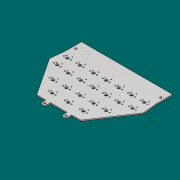
# Autodesk Inventor part: pcb_v2
Saved by Autodesk Inventor 2018 (Build 220112000, 112)
## iProperties
Created: 2021-07-30
Part Number: pcb_v2
Material: アルミニウム 6061
Document SubType Name: Modeling
Designer: gisen
Density: 2.7 g/cm^3
Appearance: アルミニウム - フラット
Author: gisen
Autodesk Inventor part; units mm, degrees
(part 1 of 2)
ref_plane "YZ Plane" through (0, 0, 0) normal (1, 0, 0) x (0, 1, 0)
ref_plane "XZ Plane" through (0, 0, 0) normal (0, 1, 0) x (-1, 0, 0)
ref_plane "XY Plane" through (0, 0, 0) normal (0, 0, 1) x (1, 0, 0)
sketch "スケッチ1" plane through (0, 0, 0) normal (0, 0, 1) x (1, 0, 0)
  line L0 (8.89, 54.5206) -> (46.4896, -2.286)
  arc A0 (46.4844, -2.2894) -> (46.4948, -2.2826) centre (46.4896, -2.286) ccw
  arc A1 (8.8952, 54.524) -> (8.8848, 54.5171) centre (8.89, 54.5206) ccw
  line L1 (150.2689, 54.5206) -> (112.6693, -2.286)
  arc A2 (112.6641, -2.2826) -> (112.6745, -2.2894) centre (112.6693, -2.286) ccw
  arc A3 (150.2742, 54.5171) -> (150.2637, 54.524) centre (150.269, 54.5206) ccw
  line L2 (147.988, 100.33) -> (11.1709, 100.33)
  arc A4 (11.1709, 100.3362) -> (11.1709, 100.3238) centre (11.1709, 100.33) ccw
  arc A5 (147.988, 100.3238) -> (147.988, 100.3362) centre (147.988, 100.33) ccw
  line L3 (11.1709, 100.33) -> (11.1709, 76.8708)
  arc A6 (11.1647, 76.8708) -> (11.1772, 76.8708) centre (11.1709, 76.8708) ccw
  arc A7 (11.1772, 100.33) -> (11.1647, 100.33) centre (11.1709, 100.33) ccw
  line L4 (8.89, 54.5206) -> (11.1709, 76.8708)
  arc A8 (11.1771, 76.8701) -> (11.1647, 76.8714) centre (11.1709, 76.8707) ccw
  arc A9 (8.8838, 54.5212) -> (8.8962, 54.5199) centre (8.89, 54.5206) ccw
  line L5 (150.2689, 54.5206) -> (147.988, 76.8708)
  arc A10 (147.9942, 76.8714) -> (147.9818, 76.8701) centre (147.988, 76.8707) ccw
  arc A11 (150.2627, 54.5199) -> (150.2752, 54.5212) centre (150.269, 54.5206) ccw
  line L6 (147.988, 100.33) -> (147.988, 76.8708)
  arc A12 (147.9818, 76.8708) -> (147.9943, 76.8708) centre (147.988, 76.8708) ccw
  arc A13 (147.9943, 100.33) -> (147.9818, 100.33) centre (147.988, 100.33) ccw
  line L7 (147.988, 76.8708) -> (150.2689, 54.5435)
  arc A14 (150.2627, 54.5428) -> (150.2752, 54.5441) centre (150.269, 54.5434) ccw
  arc A15 (147.9942, 76.8714) -> (147.9818, 76.8701) centre (147.988, 76.8707) ccw
  line L8 (46.4896, -2.286) -> (60.1294, -2.286)
  arc A16 (60.1294, -2.2923) -> (60.1294, -2.2797) centre (60.1294, -2.286) ccw
  arc A17 (46.4896, -2.2797) -> (46.4896, -2.2923) centre (46.4896, -2.286) ccw
  line L9 (67.1017, -2.286) -> (92.0572, -2.286)
  arc A18 (92.0572, -2.2923) -> (92.0572, -2.2797) centre (92.0572, -2.286) ccw
  arc A19 (67.1017, -2.2797) -> (67.1017, -2.2923) centre (67.1017, -2.286) ccw
  line L10 (99.0295, -2.286) -> (112.6693, -2.286)
  arc A20 (112.6693, -2.2923) -> (112.6693, -2.2797) centre (112.6693, -2.286) ccw
  arc A21 (99.0295, -2.2797) -> (99.0295, -2.2923) centre (99.0295, -2.286) ccw
  line L11 (67.1017, -2.286) -> (67.1017, -7.474)
  arc A22 (67.0955, -7.474) -> (67.108, -7.474) centre (67.1018, -7.474) ccw
  arc A23 (67.108, -2.286) -> (67.0955, -2.286) centre (67.1018, -2.286) ccw
  line L12 (60.1294, -2.286) -> (60.1294, -7.474)
  arc A24 (60.1232, -7.474) -> (60.1357, -7.474) centre (60.1295, -7.474) ccw
  arc A25 (60.1357, -2.286) -> (60.1232, -2.286) centre (60.1295, -2.286) ccw
  line L13 (92.0572, -2.286) -> (92.0572, -7.474)
  arc A26 (92.051, -7.474) -> (92.0635, -7.474) centre (92.0573, -7.474) ccw
  arc A27 (92.0635, -2.286) -> (92.051, -2.286) centre (92.0573, -2.286) ccw
  line L14 (99.0295, -2.286) -> (99.0295, -7.474)
  arc A28 (99.0233, -7.474) -> (99.0358, -7.474) centre (99.0296, -7.474) ccw
  arc A29 (99.0358, -2.286) -> (99.0233, -2.286) centre (99.0296, -2.286) ccw
  arc A30 (60.1294, -7.474) -> (67.1017, -7.474) centre (63.6155, -7.474) ccw
  arc A31 (60.1357, -7.474) -> (60.1232, -7.474) centre (60.1295, -7.474) ccw
  arc A32 (67.108, -7.474) -> (67.0955, -7.474) centre (67.1018, -7.474) ccw
  arc A33 (92.0572, -7.474) -> (99.0295, -7.474) centre (95.5434, -7.474) ccw
  arc A34 (92.0635, -7.474) -> (92.051, -7.474) centre (92.0573, -7.474) ccw
  arc A35 (99.0358, -7.474) -> (99.0233, -7.474) centre (99.0296, -7.474) ccw
  arc A36 (143.3652, 85.6742) -> (143.3652, 88.7222) centre (143.3652, 87.1982) ccw
  arc A37 (143.3652, 88.7222) -> (143.3652, 85.6742) centre (143.3652, 87.1982) ccw
  arc A38 (15.7937, 85.6742) -> (15.7937, 88.7222) centre (15.7937, 87.1982) ccw
  arc A39 (15.7937, 88.7222) -> (15.7937, 85.6742) centre (15.7937, 87.1982) ccw
  arc A40 (63.6156, -8.998) -> (63.6156, -5.95) centre (63.6156, -7.474) ccw
  arc A41 (63.6156, -5.95) -> (63.6156, -8.998) centre (63.6156, -7.474) ccw
  arc A42 (95.5434, -8.998) -> (95.5434, -5.95) centre (95.5434, -7.474) ccw
  arc A43 (95.5434, -5.95) -> (95.5434, -8.998) centre (95.5434, -7.474) ccw
  circle A44 centre (16.51, 68.58) radius 0.85
  circle A45 centre (26.67, 68.58) radius 0.85
  circle A46 centre (21.59, 68.58) radius 2.05
  circle A47 centre (35.56, 68.58) radius 0.85
  circle A48 centre (45.72, 68.58) radius 0.85
  circle A49 centre (40.64, 68.58) radius 2.05
  circle A50 centre (55.88, 68.58) radius 0.85
  circle A51 centre (66.04, 68.58) radius 0.85
  circle A52 centre (60.96, 68.58) radius 2.05
  circle A53 centre (74.93, 68.58) radius 0.85
  circle A54 centre (85.09, 68.58) radius 0.85
  circle A55 centre (80.01, 68.58) radius 2.05
  circle A56 centre (93.98, 68.58) radius 0.85
  circle A57 centre (104.14, 68.58) radius 0.85
  circle A58 centre (99.06, 68.58) radius 2.05
  circle A59 centre (113.03, 68.58) radius 0.85
  circle A60 centre (123.19, 68.58) radius 0.85
  circle A61 centre (118.11, 68.58) radius 2.05
  circle A62 centre (132.08, 68.58) radius 0.85
  circle A63 centre (142.24, 68.58) radius 0.85
  circle A64 centre (137.16, 68.58) radius 2.05
  circle A65 centre (17.78, 52.07) radius 0.85
  circle A66 centre (27.94, 52.07) radius 0.85
  circle A67 centre (22.86, 52.07) radius 2.05
  circle A68 centre (36.83, 49.53) radius 0.85
  circle A69 centre (46.99, 49.53) radius 0.85
  circle A70 centre (41.91, 49.53) radius 2.05
  circle A71 centre (55.88, 49.53) radius 0.85
  circle A72 centre (66.04, 49.53) radius 0.85
  circle A73 centre (60.96, 49.53) radius 2.05
  circle A74 centre (74.93, 49.53) radius 0.85
  circle A75 centre (85.09, 49.53) radius 0.85
  circle A76 centre (80.01, 49.53) radius 2.05
  circle A77 centre (93.98, 49.53) radius 0.85
  circle A78 centre (104.14, 49.53) radius 0.85
  circle A79 centre (99.06, 49.53) radius 2.05
  circle A80 centre (113.03, 49.53) radius 0.85
  circle A81 centre (123.19, 49.53) radius 0.85
  circle A82 centre (118.11, 49.53) radius 2.05
  circle A83 centre (130.81, 52.07) radius 0.85
  circle A84 centre (140.97, 52.07) radius 0.85
  circle A85 centre (135.89, 52.07) radius 2.05
  circle A86 centre (34.29, 29.21) radius 0.85
  circle A87 centre (44.45, 29.21) radius 0.85
  circle A88 centre (39.37, 29.21) radius 2.05
  circle A89 centre (54.61, 29.21) radius 0.85
  circle A90 centre (64.77, 29.21) radius 0.85
  circle A91 centre (59.69, 29.21) radius 2.05
  circle A92 centre (74.93, 29.21) radius 0.85
  circle A93 centre (85.09, 29.21) radius 0.85
  circle A94 centre (80.01, 29.21) radius 2.05
  circle A95 centre (95.25, 29.21) radius 0.85
  circle A96 centre (105.41, 29.21) radius 0.85
  circle A97 centre (100.33, 29.21) radius 2.05
  circle A98 centre (114.3, 29.21) radius 0.85
  circle A99 centre (124.46, 29.21) radius 0.85
  circle A100 centre (119.38, 29.21) radius 2.05
  circle A101 centre (50.8, 11.43) radius 0.85
  circle A102 centre (60.96, 11.43) radius 0.85
  circle A103 centre (55.88, 11.43) radius 2.05
  circle A104 centre (74.93, 11.43) radius 0.85
  circle A105 centre (85.09, 11.43) radius 0.85
  circle A106 centre (80.01, 11.43) radius 2.05
  circle A107 centre (97.79, 11.43) radius 0.85
  circle A108 centre (107.95, 11.43) radius 0.85
  circle A109 centre (102.87, 11.43) radius 2.05
  arc A110 (17.78, 70.485) -> (17.78, 71.755) centre (17.78, 71.12) ccw
  arc A111 (17.78, 71.755) -> (17.78, 70.485) centre (17.78, 71.12) ccw
  arc A112 (17.78, 70.485) -> (17.78, 71.755) centre (17.78, 71.12) ccw
  arc A113 (17.78, 71.755) -> (17.78, 70.485) centre (17.78, 71.12) ccw
  arc A114 (24.13, 73.025) -> (24.13, 74.295) centre (24.13, 73.66) ccw
  arc A115 (24.13, 74.295) -> (24.13, 73.025) centre (24.13, 73.66) ccw
  arc A116 (24.13, 73.025) -> (24.13, 74.295) centre (24.13, 73.66) ccw
  arc A117 (24.13, 74.295) -> (24.13, 73.025) centre (24.13, 73.66) ccw
  arc A118 (36.83, 70.485) -> (36.83, 71.755) centre (36.83, 71.12) ccw
  arc A119 (36.83, 71.755) -> (36.83, 70.485) centre (36.83, 71.12) ccw
  arc A120 (36.83, 70.485) -> (36.83, 71.755) centre (36.83, 71.12) ccw
  arc A121 (36.83, 71.755) -> (36.83, 70.485) centre (36.83, 71.12) ccw
  arc A122 (43.18, 73.025) -> (43.18, 74.295) centre (43.18, 73.66) ccw
  arc A123 (43.18, 74.295) -> (43.18, 73.025) centre (43.18, 73.66) ccw
  arc A124 (43.18, 73.025) -> (43.18, 74.295) centre (43.18, 73.66) ccw
  arc A125 (43.18, 74.295) -> (43.18, 73.025) centre (43.18, 73.66) ccw
  arc A126 (57.15, 70.485) -> (57.15, 71.755) centre (57.15, 71.12) ccw
  arc A127 (57.15, 71.755) -> (57.15, 70.485) centre (57.15, 71.12) ccw
  arc A128 (57.15, 70.485) -> (57.15, 71.755) centre (57.15, 71.12) ccw
  arc A129 (57.15, 71.755) -> (57.15, 70.485) centre (57.15, 71.12) ccw
  arc A130 (63.5, 73.025) -> (63.5, 74.295) centre (63.5, 73.66) ccw
  arc A131 (63.5, 74.295) -> (63.5, 73.025) centre (63.5, 73.66) ccw
  arc A132 (63.5, 73.025) -> (63.5, 74.295) centre (63.5, 73.66) ccw
  arc A133 (63.5, 74.295) -> (63.5, 73.025) centre (63.5, 73.66) ccw
  arc A134 (76.2, 70.485) -> (76.2, 71.755) centre (76.2, 71.12) ccw
  arc A135 (76.2, 71.755) -> (76.2, 70.485) centre (76.2, 71.12) ccw
  arc A136 (76.2, 70.485) -> (76.2, 71.755) centre (76.2, 71.12) ccw
  arc A137 (76.2, 71.755) -> (76.2, 70.485) centre (76.2, 71.12) ccw
  arc A138 (82.55, 73.025) -> (82.55, 74.295) centre (82.55, 73.66) ccw
  arc A139 (82.55, 74.295) -> (82.55, 73.025) centre (82.55, 73.66) ccw
  arc A140 (82.55, 73.025) -> (82.55, 74.295) centre (82.55, 73.66) ccw
  arc A141 (82.55, 74.295) -> (82.55, 73.025) centre (82.55, 73.66) ccw
  arc A142 (95.25, 70.485) -> (95.25, 71.755) centre (95.25, 71.12) ccw
  arc A143 (95.25, 71.755) -> (95.25, 70.485) centre (95.25, 71.12) ccw
  arc A144 (95.25, 70.485) -> (95.25, 71.755) centre (95.25, 71.12) ccw
  arc A145 (95.25, 71.755) -> (95.25, 70.485) centre (95.25, 71.12) ccw
  arc A146 (101.6, 73.025) -> (101.6, 74.295) centre (101.6, 73.66) ccw
  arc A147 (101.6, 74.295) -> (101.6, 73.025) centre (101.6, 73.66) ccw
  arc A148 (101.6, 73.025) -> (101.6, 74.295) centre (101.6, 73.66) ccw
  arc A149 (101.6, 74.295) -> (101.6, 73.025) centre (101.6, 73.66) ccw
  arc A150 (114.3, 70.485) -> (114.3, 71.755) centre (114.3, 71.12) ccw
  arc A151 (114.3, 71.755) -> (114.3, 70.485) centre (114.3, 71.12) ccw
  arc A152 (114.3, 70.485) -> (114.3, 71.755) centre (114.3, 71.12) ccw
  arc A153 (114.3, 71.755) -> (114.3, 70.485) centre (114.3, 71.12) ccw
  arc A154 (120.65, 73.025) -> (120.65, 74.295) centre (120.65, 73.66) ccw
  arc A155 (120.65, 74.295) -> (120.65, 73.025) centre (120.65, 73.66) ccw
  arc A156 (120.65, 73.025) -> (120.65, 74.295) centre (120.65, 73.66) ccw
  arc A157 (120.65, 74.295) -> (120.65, 73.025) centre (120.65, 73.66) ccw
  arc A158 (133.35, 70.485) -> (133.35, 71.755) centre (133.35, 71.12) ccw
  arc A159 (133.35, 71.755) -> (133.35, 70.485) centre (133.35, 71.12) ccw
  arc A160 (133.35, 70.485) -> (133.35, 71.755) centre (133.35, 71.12) ccw
  arc A161 (133.35, 71.755) -> (133.35, 70.485) centre (133.35, 71.12) ccw
  arc A162 (139.7, 73.025) -> (139.7, 74.295) centre (139.7, 73.66) ccw
  arc A163 (139.7, 74.295) -> (139.7, 73.025) centre (139.7, 73.66) ccw
  arc A164 (139.7, 73.025) -> (139.7, 74.295) centre (139.7, 73.66) ccw
  arc A165 (139.7, 74.295) -> (139.7, 73.025) centre (139.7, 73.66) ccw
  arc A166 (19.05, 53.975) -> (19.05, 55.245) centre (19.05, 54.61) ccw
  arc A167 (19.05, 55.245) -> (19.05, 53.975) centre (19.05, 54.61) ccw
  arc A168 (19.05, 53.975) -> (19.05, 55.245) centre (19.05, 54.61) ccw
  arc A169 (19.05, 55.245) -> (19.05, 53.975) centre (19.05, 54.61) ccw
  arc A170 (25.4, 56.515) -> (25.4, 57.785) centre (25.4, 57.15) ccw
  arc A171 (25.4, 57.785) -> (25.4, 56.515) centre (25.4, 57.15) ccw
  arc A172 (25.4, 56.515) -> (25.4, 57.785) centre (25.4, 57.15) ccw
  arc A173 (25.4, 57.785) -> (25.4, 56.515) centre (25.4, 57.15) ccw
  arc A174 (38.1, 51.435) -> (38.1, 52.705) centre (38.1, 52.07) ccw
  arc A175 (38.1, 52.705) -> (38.1, 51.435) centre (38.1, 52.07) ccw
  arc A176 (38.1, 51.435) -> (38.1, 52.705) centre (38.1, 52.07) ccw
  arc A177 (38.1, 52.705) -> (38.1, 51.435) centre (38.1, 52.07) ccw
  arc A178 (44.45, 53.975) -> (44.45, 55.245) centre (44.45, 54.61) ccw
  arc A179 (44.45, 55.245) -> (44.45, 53.975) centre (44.45, 54.61) ccw
  arc A180 (44.45, 53.975) -> (44.45, 55.245) centre (44.45, 54.61) ccw
  arc A181 (44.45, 55.245) -> (44.45, 53.975) centre (44.45, 54.61) ccw
  arc A182 (57.15, 51.435) -> (57.15, 52.705) centre (57.15, 52.07) ccw
  arc A183 (57.15, 52.705) -> (57.15, 51.435) centre (57.15, 52.07) ccw
  arc A184 (57.15, 51.435) -> (57.15, 52.705) centre (57.15, 52.07) ccw
  arc A185 (57.15, 52.705) -> (57.15, 51.435) centre (57.15, 52.07) ccw
  arc A186 (63.5, 53.975) -> (63.5, 55.245) centre (63.5, 54.61) ccw
  arc A187 (63.5, 55.245) -> (63.5, 53.975) centre (63.5, 54.61) ccw
  arc A188 (63.5, 53.975) -> (63.5, 55.245) centre (63.5, 54.61) ccw
  arc A189 (63.5, 55.245) -> (63.5, 53.975) centre (63.5, 54.61) ccw
  arc A190 (76.2, 51.435) -> (76.2, 52.705) centre (76.2, 52.07) ccw
  arc A191 (76.2, 52.705) -> (76.2, 51.435) centre (76.2, 52.07) ccw
  arc A192 (76.2, 51.435) -> (76.2, 52.705) centre (76.2, 52.07) ccw
  arc A193 (76.2, 52.705) -> (76.2, 51.435) centre (76.2, 52.07) ccw
  arc A194 (82.55, 53.975) -> (82.55, 55.245) centre (82.55, 54.61) ccw
  arc A195 (82.55, 55.245) -> (82.55, 53.975) centre (82.55, 54.61) ccw
  arc A196 (82.55, 53.975) -> (82.55, 55.245) centre (82.55, 54.61) ccw
  arc A197 (82.55, 55.245) -> (82.55, 53.975) centre (82.55, 54.61) ccw
  arc A198 (95.25, 51.435) -> (95.25, 52.705) centre (95.25, 52.07) ccw
  arc A199 (95.25, 52.705) -> (95.25, 51.435) centre (95.25, 52.07) ccw
  arc A200 (95.25, 51.435) -> (95.25, 52.705) centre (95.25, 52.07) ccw
  arc A201 (95.25, 52.705) -> (95.25, 51.435) centre (95.25, 52.07) ccw
  arc A202 (101.6, 53.975) -> (101.6, 55.245) centre (101.6, 54.61) ccw
  arc A203 (101.6, 55.245) -> (101.6, 53.975) centre (101.6, 54.61) ccw
  arc A204 (101.6, 53.975) -> (101.6, 55.245) centre (101.6, 54.61) ccw
  arc A205 (101.6, 55.245) -> (101.6, 53.975) centre (101.6, 54.61) ccw
  arc A206 (114.3, 51.435) -> (114.3, 52.705) centre (114.3, 52.07) ccw
  arc A207 (114.3, 52.705) -> (114.3, 51.435) centre (114.3, 52.07) ccw
  arc A208 (114.3, 51.435) -> (114.3, 52.705) centre (114.3, 52.07) ccw
  arc A209 (114.3, 52.705) -> (114.3, 51.435) centre (114.3, 52.07) ccw
  arc A210 (120.65, 53.975) -> (120.65, 55.245) centre (120.65, 54.61) ccw
  arc A211 (120.65, 55.245) -> (120.65, 53.975) centre (120.65, 54.61) ccw
  arc A212 (120.65, 53.975) -> (120.65, 55.245) centre (120.65, 54.61) ccw
  arc A213 (120.65, 55.245) -> (120.65, 53.975) centre (120.65, 54.61) ccw
  arc A214 (132.08, 53.975) -> (132.08, 55.245) centre (132.08, 54.61) ccw
  arc A215 (132.08, 55.245) -> (132.08, 53.975) centre (132.08, 54.61) ccw
  arc A216 (132.08, 53.975) -> (132.08, 55.245) centre (132.08, 54.61) ccw
  arc A217 (132.08, 55.245) -> (132.08, 53.975) centre (132.08, 54.61) ccw
  arc A218 (138.43, 56.515) -> (138.43, 57.785) centre (138.43, 57.15) ccw
  arc A219 (138.43, 57.785) -> (138.43, 56.515) centre (138.43, 57.15) ccw
  arc A220 (138.43, 56.515) -> (138.43, 57.785) centre (138.43, 57.15) ccw
  arc A221 (138.43, 57.785) -> (138.43, 56.515) centre (138.43, 57.15) ccw
  arc A222 (35.56, 31.115) -> (35.56, 32.385) centre (35.56, 31.75) ccw
  arc A223 (35.56, 32.385) -> (35.56, 31.115) centre (35.56, 31.75) ccw
  arc A224 (35.56, 31.115) -> (35.56, 32.385) centre (35.56, 31.75) ccw
  arc A225 (35.56, 32.385) -> (35.56, 31.115) centre (35.56, 31.75) ccw
  arc A226 (41.91, 33.655) -> (41.91, 34.925) centre (41.91, 34.29) ccw
  arc A227 (41.91, 34.925) -> (41.91, 33.655) centre (41.91, 34.29) ccw
  arc A228 (41.91, 33.655) -> (41.91, 34.925) centre (41.91, 34.29) ccw
  arc A229 (41.91, 34.925) -> (41.91, 33.655) centre (41.91, 34.29) ccw
  arc A230 (55.88, 31.115) -> (55.88, 32.385) centre (55.88, 31.75) ccw
  arc A231 (55.88, 32.385) -> (55.88, 31.115) centre (55.88, 31.75) ccw
  arc A232 (55.88, 31.115) -> (55.88, 32.385) centre (55.88, 31.75) ccw
  arc A233 (55.88, 32.385) -> (55.88, 31.115) centre (55.88, 31.75) ccw
  arc A234 (62.23, 33.655) -> (62.23, 34.925) centre (62.23, 34.29) ccw
  arc A235 (62.23, 34.925) -> (62.23, 33.655) centre (62.23, 34.29) ccw
  arc A236 (62.23, 33.655) -> (62.23, 34.925) centre (62.23, 34.29) ccw
  arc A237 (62.23, 34.925) -> (62.23, 33.655) centre (62.23, 34.29) ccw
  arc A238 (76.2, 31.115) -> (76.2, 32.385) centre (76.2, 31.75) ccw
  arc A239 (76.2, 32.385) -> (76.2, 31.115) centre (76.2, 31.75) ccw
  arc A240 (76.2, 31.115) -> (76.2, 32.385) centre (76.2, 31.75) ccw
  arc A241 (76.2, 32.385) -> (76.2, 31.115) centre (76.2, 31.75) ccw
  arc A242 (82.55, 33.655) -> (82.55, 34.925) centre (82.55, 34.29) ccw
  arc A243 (82.55, 34.925) -> (82.55, 33.655) centre (82.55, 34.29) ccw
  arc A244 (82.55, 33.655) -> (82.55, 34.925) centre (82.55, 34.29) ccw
  arc A245 (82.55, 34.925) -> (82.55, 33.655) centre (82.55, 34.29) ccw
  arc A246 (96.52, 31.115) -> (96.52, 32.385) centre (96.52, 31.75) ccw
  arc A247 (96.52, 32.385) -> (96.52, 31.115) centre (96.52, 31.75) ccw
  arc A248 (96.52, 31.115) -> (96.52, 32.385) centre (96.52, 31.75) ccw
  arc A249 (96.52, 32.385) -> (96.52, 31.115) centre (96.52, 31.75) ccw
  arc A250 (102.87, 33.655) -> (102.87, 34.925) centre (102.87, 34.29) ccw
  arc A251 (102.87, 34.925) -> (102.87, 33.655) centre (102.87, 34.29) ccw
  arc A252 (102.87, 33.655) -> (102.87, 34.925) centre (102.87, 34.29) ccw
  arc A253 (102.87, 34.925) -> (102.87, 33.655) centre (102.87, 34.29) ccw
  arc A254 (115.57, 31.115) -> (115.57, 32.385) centre (115.57, 31.75) ccw
  arc A255 (115.57, 32.385) -> (115.57, 31.115) centre (115.57, 31.75) ccw
  arc A256 (115.57, 31.115) -> (115.57, 32.385) centre (115.57, 31.75) ccw
  arc A257 (115.57, 32.385) -> (115.57, 31.115) centre (115.57, 31.75) ccw
  arc A258 (121.92, 33.655) -> (121.92, 34.925) centre (121.92, 34.29) ccw
  arc A259 (121.92, 34.925) -> (121.92, 33.655) centre (121.92, 34.29) ccw
  arc A260 (121.92, 33.655) -> (121.92, 34.925) centre (121.92, 34.29) ccw
  arc A261 (121.92, 34.925) -> (121.92, 33.655) centre (121.92, 34.29) ccw
  arc A262 (52.07, 13.335) -> (52.07, 14.605) centre (52.07, 13.97) ccw
  arc A263 (52.07, 14.605) -> (52.07, 13.335) centre (52.07, 13.97) ccw
  arc A264 (52.07, 13.335) -> (52.07, 14.605) centre (52.07, 13.97) ccw
  arc A265 (52.07, 14.605) -> (52.07, 13.335) centre (52.07, 13.97) ccw
  arc A266 (58.42, 15.875) -> (58.42, 17.145) centre (58.42, 16.51) ccw
  arc A267 (58.42, 17.145) -> (58.42, 15.875) centre (58.42, 16.51) ccw
  arc A268 (58.42, 15.875) -> (58.42, 17.145) centre (58.42, 16.51) ccw
  arc A269 (58.42, 17.145) -> (58.42, 15.875) centre (58.42, 16.51) ccw
  arc A270 (76.2, 13.335) -> (76.2, 14.605) centre (76.2, 13.97) ccw
  arc A271 (76.2, 14.605) -> (76.2, 13.335) centre (76.2, 13.97) ccw
  arc A272 (76.2, 13.335) -> (76.2, 14.605) centre (76.2, 13.97) ccw
  arc A273 (76.2, 14.605) -> (76.2, 13.335) centre (76.2, 13.97) ccw
  arc A274 (82.55, 15.875) -> (82.55, 17.145) centre (82.55, 16.51) ccw
  arc A275 (82.55, 17.145) -> (82.55, 15.875) centre (82.55, 16.51) ccw
  arc A276 (82.55, 15.875) -> (82.55, 17.145) centre (82.55, 16.51) ccw
  arc A277 (82.55, 17.145) -> (82.55, 15.875) centre (82.55, 16.51) ccw
  arc A278 (99.06, 13.335) -> (99.06, 14.605) centre (99.06, 13.97) ccw
  arc A279 (99.06, 14.605) -> (99.06, 13.335) centre (99.06, 13.97) ccw
  arc A280 (99.06, 13.335) -> (99.06, 14.605) centre (99.06, 13.97) ccw
  arc A281 (99.06, 14.605) -> (99.06, 13.335) centre (99.06, 13.97) ccw
  arc A282 (105.41, 15.875) -> (105.41, 17.145) centre (105.41, 16.51) ccw
  arc A283 (105.41, 17.145) -> (105.41, 15.875) centre (105.41, 16.51) ccw
  arc A284 (105.41, 15.875) -> (105.41, 17.145) centre (105.41, 16.51) ccw
  arc A285 (105.41, 17.145) -> (105.41, 15.875) centre (105.41, 16.51) ccw
  line L15 (18.55, 99.449) -> (19.55, 99.449) construction
  line L16 (19.55, 99.449) -> (19.55, 100.449) construction
  line L17 (19.55, 100.449) -> (18.55, 100.449) construction
  line L18 (18.55, 100.449) -> (18.55, 99.449) construction
  line L19 (21.09, 99.449) -> (22.09, 99.449) construction
  line L20 (22.09, 99.449) -> (22.09, 100.449) construction
  line L21 (22.09, 100.449) -> (21.09, 100.449) construction
  line L22 (21.09, 100.449) -> (21.09, 99.449) construction
  line L23 (23.63, 99.449) -> (24.63, 99.449) construction
  line L24 (24.63, 99.449) -> (24.63, 100.449) construction
  line L25 (24.63, 100.449) -> (23.63, 100.449) construction
  line L26 (23.63, 100.449) -> (23.63, 99.449) construction
  line L27 (26.17, 99.449) -> (27.17, 99.449) construction
  line L28 (27.17, 99.449) -> (27.17, 100.449) construction
  line L29 (27.17, 100.449) -> (26.17, 100.449) construction
  line L30 (26.17, 100.449) -> (26.17, 99.449) construction
  line L31 (28.71, 99.449) -> (29.71, 99.449) construction
  line L32 (29.71, 99.449) -> (29.71, 100.449) construction
  line L33 (29.71, 100.449) -> (28.71, 100.449) construction
  line L34 (28.71, 100.449) -> (28.71, 99.449) construction
  line L35 (31.25, 99.449) -> (32.25, 99.449) construction
  line L36 (32.25, 99.449) -> (32.25, 100.449) construction
  line L37 (32.25, 100.449) -> (31.25, 100.449) construction
  line L38 (31.25, 100.449) -> (31.25, 99.449) construction
  line L39 (33.79, 99.449) -> (34.79, 99.449) construction
  line L40 (34.79, 99.449) -> (34.79, 100.449) construction
  line L41 (34.79, 100.449) -> (33.79, 100.449) construction
  line L42 (33.79, 100.449) -> (33.79, 99.449) construction
  line L43 (36.33, 99.449) -> (37.33, 99.449) construction
  line L44 (37.33, 99.449) -> (37.33, 100.449) construction
  line L45 (37.33, 100.449) -> (36.33, 100.449) construction
  line L46 (36.33, 100.449) -> (36.33, 99.449) construction
  line L47 (38.87, 99.449) -> (39.87, 99.449) construction
  line L48 (39.87, 99.449) -> (39.87, 100.449) construction
  line L49 (39.87, 100.449) -> (38.87, 100.449) construction
  line L50 (38.87, 100.449) -> (38.87, 99.449) construction
  line L51 (41.41, 99.449) -> (42.41, 99.449) construction
  line L52 (42.41, 99.449) -> (42.41, 100.449) construction
  line L53 (42.41, 100.449) -> (41.41, 100.449) construction
  line L54 (41.41, 100.449) -> (41.41, 99.449) construction
  line L55 (43.95, 99.449) -> (44.95, 99.449) construction
  line L56 (44.95, 99.449) -> (44.95, 100.449) construction
  line L57 (44.95, 100.449) -> (43.95, 100.449) construction
  line L58 (43.95, 100.449) -> (43.95, 99.449) construction
  line L59 (46.49, 99.449) -> (47.49, 99.449) construction
  line L60 (47.49, 99.449) -> (47.49, 100.449) construction
  line L61 (47.49, 100.449) -> (46.49, 100.449) construction
  line L62 (46.49, 100.449) -> (46.49, 99.449) construction
  line L63 (49.03, 99.449) -> (50.03, 99.449) construction
  line L64 (50.03, 99.449) -> (50.03, 100.449) construction
  line L65 (50.03, 100.449) -> (49.03, 100.449) construction
  line L66 (49.03, 100.449) -> (49.03, 99.449) construction
  line L67 (51.57, 99.449) -> (52.57, 99.449) construction
  line L68 (52.57, 99.449) -> (52.57, 100.449) construction
  line L69 (52.57, 100.449) -> (51.57, 100.449) construction
  line L70 (51.57, 100.449) -> (51.57, 99.449) construction
  line L71 (54.11, 99.449) -> (55.11, 99.449) construction
  line L72 (55.11, 99.449) -> (55.11, 100.449) construction
  line L73 (55.11, 100.449) -> (54.11, 100.449) construction
  line L74 (54.11, 100.449) -> (54.11, 99.449) construction
  line L75 (56.65, 99.449) -> (57.65, 99.449) construction
  line L76 (57.65, 99.449) -> (57.65, 100.449) construction
  line L77 (57.65, 100.449) -> (56.65, 100.449) construction
  line L78 (56.65, 100.449) -> (56.65, 99.449) construction
  line L79 (59.19, 99.449) -> (60.19, 99.449) construction
  line L80 (60.19, 99.449) -> (60.19, 100.449) construction
  line L81 (60.19, 100.449) -> (59.19, 100.449) construction
  line L82 (59.19, 100.449) -> (59.19, 99.449) construction
  line L83 (61.73, 99.449) -> (62.73, 99.449) construction
  line L84 (62.73, 99.449) -> (62.73, 100.449) construction
  line L85 (62.73, 100.449) -> (61.73, 100.449) construction
  line L86 (61.73, 100.449) -> (61.73, 99.449) construction
  line L87 (18.55, 96.147) -> (19.55, 96.147) construction
  line L88 (19.55, 96.147) -> (19.55, 97.147) construction
  line L89 (19.55, 97.147) -> (18.55, 97.147) construction
  line L90 (18.55, 97.147) -> (18.55, 96.147) construction
  line L91 (21.09, 96.147) -> (22.09, 96.147) construction
  line L92 (22.09, 96.147) -> (22.09, 97.147) construction
  line L93 (22.09, 97.147) -> (21.09, 97.147) construction
  line L94 (21.09, 97.147) -> (21.09, 96.147) construction
  line L95 (23.63, 96.147) -> (24.63, 96.147) construction
  line L96 (24.63, 96.147) -> (24.63, 97.147) construction
  line L97 (24.63, 97.147) -> (23.63, 97.147) construction
  line L98 (23.63, 97.147) -> (23.63, 96.147) construction
  line L99 (26.17, 96.147) -> (27.17, 96.147) construction
  line L100 (27.17, 96.147) -> (27.17, 97.147) construction
  line L101 (27.17, 97.147) -> (26.17, 97.147) construction
  line L102 (26.17, 97.147) -> (26.17, 96.147) construction
  line L103 (28.71, 96.147) -> (29.71, 96.147) construction
  line L104 (29.71, 96.147) -> (29.71, 97.147) construction
  line L105 (29.71, 97.147) -> (28.71, 97.147) construction
  line L106 (28.71, 97.147) -> (28.71, 96.147) construction
  line L107 (31.25, 96.147) -> (32.25, 96.147) construction
  line L108 (32.25, 96.147) -> (32.25, 97.147) construction
  line L109 (32.25, 97.147) -> (31.25, 97.147) construction
  line L110 (31.25, 97.147) -> (31.25, 96.147) construction
  line L111 (33.79, 96.147) -> (34.79, 96.147) construction
  line L112 (34.79, 96.147) -> (34.79, 97.147) construction
  line L113 (34.79, 97.147) -> (33.79, 97.147) construction
  line L114 (33.79, 97.147) -> (33.79, 96.147) construction
  line L115 (36.33, 96.147) -> (37.33, 96.147) construction
  line L116 (37.33, 96.147) -> (37.33, 97.147) construction
  line L117 (37.33, 97.147) -> (36.33, 97.147) construction
  line L118 (36.33, 97.147) -> (36.33, 96.147) construction
  line L119 (38.87, 96.147) -> (39.87, 96.147) construction
  line L120 (39.87, 96.147) -> (39.87, 97.147) construction
  line L121 (39.87, 97.147) -> (38.87, 97.147) construction
  line L122 (38.87, 97.147) -> (38.87, 96.147) construction
  line L123 (41.41, 96.147) -> (42.41, 96.147) construction
  line L124 (42.41, 96.147) -> (42.41, 97.147) construction
  line L125 (42.41, 97.147) -> (41.41, 97.147) construction
  line L126 (41.41, 97.147) -> (41.41, 96.147) construction
  line L127 (43.95, 96.147) -> (44.95, 96.147) construction
  line L128 (44.95, 96.147) -> (44.95, 97.147) construction
  line L129 (44.95, 97.147) -> (43.95, 97.147) construction
  line L130 (43.95, 97.147) -> (43.95, 96.147) construction
  line L131 (46.49, 96.147) -> (47.49, 96.147) construction
  line L132 (47.49, 96.147) -> (47.49, 97.147) construction
  line L133 (47.49, 97.147) -> (46.49, 97.147) construction
  line L134 (46.49, 97.147) -> (46.49, 96.147) construction
  line L135 (49.03, 96.147) -> (50.03, 96.147) construction
  line L136 (50.03, 96.147) -> (50.03, 97.147) construction
  line L137 (50.03, 97.147) -> (49.03, 97.147) construction
  line L138 (49.03, 97.147) -> (49.03, 96.147) construction
  line L139 (51.57, 96.147) -> (52.57, 96.147) construction
  line L140 (52.57, 96.147) -> (52.57, 97.147) construction
  line L141 (52.57, 97.147) -> (51.57, 97.147) construction
  line L142 (51.57, 97.147) -> (51.57, 96.147) construction
  line L143 (54.11, 96.147) -> (55.11, 96.147) construction
  line L144 (55.11, 96.147) -> (55.11, 97.147) construction
  line L145 (55.11, 97.147) -> (54.11, 97.147) construction
  line L146 (54.11, 97.147) -> (54.11, 96.147) construction
  line L147 (56.65, 96.147) -> (57.65, 96.147) construction
  line L148 (57.65, 96.147) -> (57.65, 97.147) construction
  line L149 (57.65, 97.147) -> (56.65, 97.147) construction
  line L150 (56.65, 97.147) -> (56.65, 96.147) construction
  line L151 (59.19, 96.147) -> (60.19, 96.147) construction
  line L152 (60.19, 96.147) -> (60.19, 97.147) construction
  line L153 (60.19, 97.147) -> (59.19, 97.147) construction
  line L154 (59.19, 97.147) -> (59.19, 96.147) construction
  line L155 (61.73, 96.147) -> (62.73, 96.147) construction
  line L156 (62.73, 96.147) -> (62.73, 97.147) construction
  line L157 (62.73, 97.147) -> (61.73, 97.147) construction
  line L158 (61.73, 97.147) -> (61.73, 96.147) construction
  line L159 (19.05, 94.488) -> (19.05, 96.012) construction
  arc A286 (19.431, 96.012) -> (18.669, 96.012) centre (19.05, 96.012) ccw construction
  arc A287 (18.669, 94.488) -> (19.431, 94.488) centre (19.05, 94.488) ccw construction
  line L160 (19.05, 94.488) -> (19.05, 96.012) construction
  arc A288 (19.431, 96.012) -> (18.669, 96.012) centre (19.05, 96.012) ccw construction
  arc A289 (18.669, 94.488) -> (19.431, 94.488) centre (19.05, 94.488) ccw construction
  line L161 (21.59, 94.488) -> (21.59, 96.012) construction
  arc A290 (21.971, 96.012) -> (21.209, 96.012) centre (21.59, 96.012) ccw construction
  arc A291 (21.209, 94.488) -> (21.971, 94.488) centre (21.59, 94.488) ccw construction
  line L162 (21.59, 94.488) -> (21.59, 96.012) construction
  arc A292 (21.971, 96.012) -> (21.209, 96.012) centre (21.59, 96.012) ccw construction
  arc A293 (21.209, 94.488) -> (21.971, 94.488) centre (21.59, 94.488) ccw construction
  line L163 (24.13, 94.488) -> (24.13, 96.012) construction
  arc A294 (24.511, 96.012) -> (23.749, 96.012) centre (24.13, 96.012) ccw construction
  arc A295 (23.749, 94.488) -> (24.511, 94.488) centre (24.13, 94.488) ccw construction
  line L164 (24.13, 94.488) -> (24.13, 96.012) construction
  arc A296 (24.511, 96.012) -> (23.749, 96.012) centre (24.13, 96.012) ccw construction
  arc A297 (23.749, 94.488) -> (24.511, 94.488) centre (24.13, 94.488) ccw construction
  line L165 (26.67, 94.488) -> (26.67, 96.012) construction
  arc A298 (27.051, 96.012) -> (26.289, 96.012) centre (26.67, 96.012) ccw construction
  arc A299 (26.289, 94.488) -> (27.051, 94.488) centre (26.67, 94.488) ccw construction
  line L166 (26.67, 94.488) -> (26.67, 96.012) construction
  arc A300 (27.051, 96.012) -> (26.289, 96.012) centre (26.67, 96.012) ccw construction
  arc A301 (26.289, 94.488) -> (27.051, 94.488) centre (26.67, 94.488) ccw construction
  line L167 (29.21, 94.488) -> (29.21, 96.012) construction
  arc A302 (29.591, 96.012) -> (28.829, 96.012) centre (29.21, 96.012) ccw construction
  arc A303 (28.829, 94.488) -> (29.591, 94.488) centre (29.21, 94.488) ccw construction
  line L168 (29.21, 94.488) -> (29.21, 96.012) construction
  arc A304 (29.591, 96.012) -> (28.829, 96.012) centre (29.21, 96.012) ccw construction
  arc A305 (28.829, 94.488) -> (29.591, 94.488) centre (29.21, 94.488) ccw construction
  line L169 (31.75, 94.488) -> (31.75, 96.012) construction
  arc A306 (32.131, 96.012) -> (31.369, 96.012) centre (31.75, 96.012) ccw construction
  arc A307 (31.369, 94.488) -> (32.131, 94.488) centre (31.75, 94.488) ccw construction
  line L170 (31.75, 94.488) -> (31.75, 96.012) construction
  arc A308 (32.131, 96.012) -> (31.369, 96.012) centre (31.75, 96.012) ccw construction
  arc A309 (31.369, 94.488) -> (32.131, 94.488) centre (31.75, 94.488) ccw construction
  line L171 (34.29, 94.488) -> (34.29, 96.012) construction
  arc A310 (34.671, 96.012) -> (33.909, 96.012) centre (34.29, 96.012) ccw construction
  arc A311 (33.909, 94.488) -> (34.671, 94.488) centre (34.29, 94.488) ccw construction
  line L172 (34.29, 94.488) -> (34.29, 96.012) construction
  arc A312 (34.671, 96.012) -> (33.909, 96.012) centre (34.29, 96.012) ccw construction
  arc A313 (33.909, 94.488) -> (34.671, 94.488) centre (34.29, 94.488) ccw construction
  line L173 (36.83, 94.488) -> (36.83, 96.012) construction
  arc A314 (37.211, 96.012) -> (36.449, 96.012) centre (36.83, 96.012) ccw construction
  arc A315 (36.449, 94.488) -> (37.211, 94.488) centre (36.83, 94.488) ccw construction
  line L174 (36.83, 94.488) -> (36.83, 96.012) construction
  arc A316 (37.211, 96.012) -> (36.449, 96.012) centre (36.83, 96.012) ccw construction
  arc A317 (36.449, 94.488) -> (37.211, 94.488) centre (36.83, 94.488) ccw construction
  line L175 (39.37, 94.488) -> (39.37, 96.012) construction
  arc A318 (39.751, 96.012) -> (38.989, 96.012) centre (39.37, 96.012) ccw construction
  arc A319 (38.989, 94.488) -> (39.751, 94.488) centre (39.37, 94.488) ccw construction
  line L176 (39.37, 94.488) -> (39.37, 96.012) construction
  arc A320 (39.751, 96.012) -> (38.989, 96.012) centre (39.37, 96.012) ccw construction
  arc A321 (38.989, 94.488) -> (39.751, 94.488) centre (39.37, 94.488) ccw construction
  line L177 (41.91, 94.488) -> (41.91, 96.012) construction
  arc A322 (42.291, 96.012) -> (41.529, 96.012) centre (41.91, 96.012) ccw construction
  arc A323 (41.529, 94.488) -> (42.291, 94.488) centre (41.91, 94.488) ccw construction
  line L178 (41.91, 94.488) -> (41.91, 96.012) construction
  arc A324 (42.291, 96.012) -> (41.529, 96.012) centre (41.91, 96.012) ccw construction
  arc A325 (41.529, 94.488) -> (42.291, 94.488) centre (41.91, 94.488) ccw construction
  line L179 (44.45, 94.488) -> (44.45, 96.012) construction
  arc A326 (44.831, 96.012) -> (44.069, 96.012) centre (44.45, 96.012) ccw construction
  arc A327 (44.069, 94.488) -> (44.831, 94.488) centre (44.45, 94.488) ccw construction
  line L180 (44.45, 94.488) -> (44.45, 96.012) construction
  arc A328 (44.831, 96.012) -> (44.069, 96.012) centre (44.45, 96.012) ccw construction
  arc A329 (44.069, 94.488) -> (44.831, 94.488) centre (44.45, 94.488) ccw construction
  line L181 (46.99, 94.488) -> (46.99, 96.012) construction
  arc A330 (47.371, 96.012) -> (46.609, 96.012) centre (46.99, 96.012) ccw construction
  arc A331 (46.609, 94.488) -> (47.371, 94.488) centre (46.99, 94.488) ccw construction
  line L182 (46.99, 94.488) -> (46.99, 96.012) construction
  arc A332 (47.371, 96.012) -> (46.609, 96.012) centre (46.99, 96.012) ccw construction
  arc A333 (46.609, 94.488) -> (47.371, 94.488) centre (46.99, 94.488) ccw construction
  line L183 (49.53, 94.488) -> (49.53, 96.012) construction
  arc A334 (49.911, 96.012) -> (49.149, 96.012) centre (49.53, 96.012) ccw construction
  arc A335 (49.149, 94.488) -> (49.911, 94.488) centre (49.53, 94.488) ccw construction
  line L184 (49.53, 94.488) -> (49.53, 96.012) construction
  arc A336 (49.911, 96.012) -> (49.149, 96.012) centre (49.53, 96.012) ccw construction
  arc A337 (49.149, 94.488) -> (49.911, 94.488) centre (49.53, 94.488) ccw construction
  line L185 (52.07, 94.488) -> (52.07, 96.012) construction
  arc A338 (52.451, 96.012) -> (51.689, 96.012) centre (52.07, 96.012) ccw construction
  arc A339 (51.689, 94.488) -> (52.451, 94.488) centre (52.07, 94.488) ccw construction
  line L186 (52.07, 94.488) -> (52.07, 96.012) construction
  arc A340 (52.451, 96.012) -> (51.689, 96.012) centre (52.07, 96.012) ccw construction
  arc A341 (51.689, 94.488) -> (52.451, 94.488) centre (52.07, 94.488) ccw construction
  line L187 (54.61, 94.488) -> (54.61, 96.012) construction
  arc A342 (54.991, 96.012) -> (54.229, 96.012) centre (54.61, 96.012) ccw construction
  arc A343 (54.229, 94.488) -> (54.991, 94.488) centre (54.61, 94.488) ccw construction
  line L188 (54.61, 94.488) -> (54.61, 96.012) construction
  arc A344 (54.991, 96.012) -> (54.229, 96.012) centre (54.61, 96.012) ccw construction
  arc A345 (54.229, 94.488) -> (54.991, 94.488) centre (54.61, 94.488) ccw construction
  line L189 (57.15, 94.488) -> (57.15, 96.012) construction
  arc A346 (57.531, 96.012) -> (56.769, 96.012) centre (57.15, 96.012) ccw construction
  arc A347 (56.769, 94.488) -> (57.531, 94.488) centre (57.15, 94.488) ccw construction
  line L190 (57.15, 94.488) -> (57.15, 96.012) construction
  arc A348 (57.531, 96.012) -> (56.769, 96.012) centre (57.15, 96.012) ccw construction
  arc A349 (56.769, 94.488) -> (57.531, 94.488) centre (57.15, 94.488) ccw construction
  line L191 (59.69, 94.488) -> (59.69, 96.012) construction
  arc A350 (60.071, 96.012) -> (59.309, 96.012) centre (59.69, 96.012) ccw construction
  arc A351 (59.309, 94.488) -> (60.071, 94.488) centre (59.69, 94.488) ccw construction
  line L192 (59.69, 94.488) -> (59.69, 96.012) construction
  arc A352 (60.071, 96.012) -> (59.309, 96.012) centre (59.69, 96.012) ccw construction
  arc A353 (59.309, 94.488) -> (60.071, 94.488) centre (59.69, 94.488) ccw construction
  line L193 (62.23, 94.488) -> (62.23, 96.012) construction
  arc A354 (62.611, 96.012) -> (61.849, 96.012) centre (62.23, 96.012) ccw construction
  arc A355 (61.849, 94.488) -> (62.611, 94.488) centre (62.23, 94.488) ccw construction
  line L194 (62.23, 94.488) -> (62.23, 96.012) construction
  arc A356 (62.611, 96.012) -> (61.849, 96.012) centre (62.23, 96.012) ccw construction
  arc A357 (61.849, 94.488) -> (62.611, 94.488) centre (62.23, 94.488) ccw construction
  line L195 (107.45, 99.449) -> (108.45, 99.449) construction
  line L196 (108.45, 99.449) -> (108.45, 100.449) construction
  line L197 (108.45, 100.449) -> (107.45, 100.449) construction
  line L198 (107.45, 100.449) -> (107.45, 99.449) construction
  line L199 (109.99, 99.449) -> (110.99, 99.449) construction
  line L200 (110.99, 99.449) -> (110.99, 100.449) construction
  line L201 (110.99, 100.449) -> (109.99, 100.449) construction
  line L202 (109.99, 100.449) -> (109.99, 99.449) construction
  line L203 (112.53, 99.449) -> (113.53, 99.449) construction
  line L204 (113.53, 99.449) -> (113.53, 100.449) construction
  line L205 (113.53, 100.449) -> (112.53, 100.449) construction
  line L206 (112.53, 100.449) -> (112.53, 99.449) construction
  line L207 (115.07, 99.449) -> (116.07, 99.449) construction
  line L208 (116.07, 99.449) -> (116.07, 100.449) construction
  line L209 (116.07, 100.449) -> (115.07, 100.449) construction
  line L210 (115.07, 100.449) -> (115.07, 99.449) construction
  line L211 (117.61, 99.449) -> (118.61, 99.449) construction
  line L212 (118.61, 99.449) -> (118.61, 100.449) construction
  line L213 (118.61, 100.449) -> (117.61, 100.449) construction
  line L214 (117.61, 100.449) -> (117.61, 99.449) construction
  line L215 (120.15, 99.449) -> (121.15, 99.449) construction
  line L216 (121.15, 99.449) -> (121.15, 100.449) construction
  line L217 (121.15, 100.449) -> (120.15, 100.449) construction
  line L218 (120.15, 100.449) -> (120.15, 99.449) construction
  line L219 (122.69, 99.449) -> (123.69, 99.449) construction
  line L220 (123.69, 99.449) -> (123.69, 100.449) construction
  line L221 (123.69, 100.449) -> (122.69, 100.449) construction
  line L222 (122.69, 100.449) -> (122.69, 99.449) construction
  line L223 (125.23, 99.449) -> (126.23, 99.449) construction
  line L224 (126.23, 99.449) -> (126.23, 100.449) construction
  line L225 (126.23, 100.449) -> (125.23, 100.449) construction
  line L226 (125.23, 100.449) -> (125.23, 99.449) construction
  line L227 (127.77, 99.449) -> (128.77, 99.449) construction
  line L228 (128.77, 99.449) -> (128.77, 100.449) construction
  line L229 (128.77, 100.449) -> (127.77, 100.449) construction
  line L230 (127.77, 100.449) -> (127.77, 99.449) construction
  line L231 (130.31, 99.449) -> (131.31, 99.449) construction
  line L232 (131.31, 99.449) -> (131.31, 100.449) construction
  line L233 (131.31, 100.449) -> (130.31, 100.449) construction
  line L234 (130.31, 100.449) -> (130.31, 99.449) construction
  line L235 (132.85, 99.449) -> (133.85, 99.449) construction
  line L236 (133.85, 99.449) -> (133.85, 100.449) construction
  line L237 (133.85, 100.449) -> (132.85, 100.449) construction
  line L238 (132.85, 100.449) -> (132.85, 99.449) construction
  line L239 (135.39, 99.449) -> (136.39, 99.449) construction
  line L240 (136.39, 99.449) -> (136.39, 100.449) construction
  line L241 (136.39, 100.449) -> (135.39, 100.449) construction
  line L242 (135.39, 100.449) -> (135.39, 99.449) construction
  line L243 (137.93, 99.449) -> (138.93, 99.449) construction
  line L244 (138.93, 99.449) -> (138.93, 100.449) construction
  line L245 (138.93, 100.449) -> (137.93, 100.449) construction
  line L246 (137.93, 100.449) -> (137.93, 99.449) construction
  line L247 (140.47, 99.449) -> (141.47, 99.449) construction
  line L248 (141.47, 99.449) -> (141.47, 100.449) construction
  line L249 (141.47, 100.449) -> (140.47, 100.449) construction
  line L250 (140.47, 100.449) -> (140.47, 99.449) construction
  line L251 (143.01, 99.449) -> (144.01, 99.449) construction
  line L252 (144.01, 99.449) -> (144.01, 100.449) construction
  line L253 (144.01, 100.449) -> (143.01, 100.449) construction
  line L254 (143.01, 100.449) -> (143.01, 99.449) construction
  line L255 (107.45, 96.147) -> (108.45, 96.147) construction
  line L256 (108.45, 96.147) -> (108.45, 97.147) construction
  line L257 (108.45, 97.147) -> (107.45, 97.147) construction
  line L258 (107.45, 97.147) -> (107.45, 96.147) construction
  line L259 (109.99, 96.147) -> (110.99, 96.147) construction
  line L260 (110.99, 96.147) -> (110.99, 97.147) construction
  line L261 (110.99, 97.147) -> (109.99, 97.147) construction
  line L262 (109.99, 97.147) -> (109.99, 96.147) construction
  line L263 (112.53, 96.147) -> (113.53, 96.147) construction
  line L264 (113.53, 96.147) -> (113.53, 97.147) construction
  line L265 (113.53, 97.147) -> (112.53, 97.147) construction
  line L266 (112.53, 97.147) -> (112.53, 96.147) construction
  line L267 (115.07, 96.147) -> (116.07, 96.147) construction
  line L268 (116.07, 96.147) -> (116.07, 97.147) construction
  line L269 (116.07, 97.147) -> (115.07, 97.147) construction
  line L270 (115.07, 97.147) -> (115.07, 96.147) construction
  line L271 (117.61, 96.147) -> (118.61, 96.147) construction
  line L272 (118.61, 96.147) -> (118.61, 97.147) construction
  line L273 (118.61, 97.147) -> (117.61, 97.147) construction
  line L274 (117.61, 97.147) -> (117.61, 96.147) construction
  line L275 (120.15, 96.147) -> (121.15, 96.147) construction
  line L276 (121.15, 96.147) -> (121.15, 97.147) construction
  line L277 (121.15, 97.147) -> (120.15, 97.147) construction
  line L278 (120.15, 97.147) -> (120.15, 96.147) construction
  line L279 (122.69, 96.147) -> (123.69, 96.147) construction
  line L280 (123.69, 96.147) -> (123.69, 97.147) construction
  line L281 (123.69, 97.147) -> (122.69, 97.147) construction
  line L282 (122.69, 97.147) -> (122.69, 96.147) construction
  line L283 (125.23, 96.147) -> (126.23, 96.147) construction
  line L284 (126.23, 96.147) -> (126.23, 97.147) construction
  line L285 (126.23, 97.147) -> (125.23, 97.147) construction
  line L286 (125.23, 97.147) -> (125.23, 96.147) construction
  line L287 (127.77, 96.147) -> (128.77, 96.147) construction
  line L288 (128.77, 96.147) -> (128.77, 97.147) construction
  line L289 (128.77, 97.147) -> (127.77, 97.147) construction
  line L290 (127.77, 97.147) -> (127.77, 96.147) construction
  line L291 (130.31, 96.147) -> (131.31, 96.147) construction
  line L292 (131.31, 96.147) -> (131.31, 97.147) construction
  line L293 (131.31, 97.147) -> (130.31, 97.147) construction
  line L294 (130.31, 97.147) -> (130.31, 96.147) construction
  line L295 (132.85, 96.147) -> (133.85, 96.147) construction
  line L296 (133.85, 96.147) -> (133.85, 97.147) construction
  line L297 (133.85, 97.147) -> (132.85, 97.147) construction
  line L298 (132.85, 97.147) -> (132.85, 96.147) construction
  line L299 (135.39, 96.147) -> (136.39, 96.147) construction
  line L300 (136.39, 96.147) -> (136.39, 97.147) construction
  line L301 (136.39, 97.147) -> (135.39, 97.147) construction
  line L302 (135.39, 97.147) -> (135.39, 96.147) construction
  line L303 (137.93, 96.147) -> (138.93, 96.147) construction
  line L304 (138.93, 96.147) -> (138.93, 97.147) construction
  line L305 (138.93, 97.147) -> (137.93, 97.147) construction
  line L306 (137.93, 97.147) -> (137.93, 96.147) construction
  line L307 (140.47, 96.147) -> (141.47, 96.147) construction
  line L308 (141.47, 96.147) -> (141.47, 97.147) construction
  line L309 (141.47, 97.147) -> (140.47, 97.147) construction
  line L310 (140.47, 97.147) -> (140.47, 96.147) construction
  line L311 (143.01, 96.147) -> (144.01, 96.147) construction
  line L312 (144.01, 96.147) -> (144.01, 97.147) construction
  line L313 (144.01, 97.147) -> (143.01, 97.147) construction
  line L314 (143.01, 97.147) -> (143.01, 96.147) construction
  line L315 (107.95, 94.488) -> (107.95, 96.012) construction
  arc A358 (108.331, 96.012) -> (107.569, 96.012) centre (107.95, 96.012) ccw construction
  arc A359 (107.569, 94.488) -> (108.331, 94.488) centre (107.95, 94.488) ccw construction
  line L316 (107.95, 94.488) -> (107.95, 96.012) construction
  arc A360 (108.331, 96.012) -> (107.569, 96.012) centre (107.95, 96.012) ccw construction
  arc A361 (107.569, 94.488) -> (108.331, 94.488) centre (107.95, 94.488) ccw construction
  line L317 (110.49, 94.488) -> (110.49, 96.012) construction
  arc A362 (110.871, 96.012) -> (110.109, 96.012) centre (110.49, 96.012) ccw construction
  arc A363 (110.109, 94.488) -> (110.871, 94.488) centre (110.49, 94.488) ccw construction
  line L318 (110.49, 94.488) -> (110.49, 96.012) construction
  arc A364 (110.871, 96.012) -> (110.109, 96.012) centre (110.49, 96.012) ccw construction
  arc A365 (110.109, 94.488) -> (110.871, 94.488) centre (110.49, 94.488) ccw construction
  line L319 (113.03, 94.488) -> (113.03, 96.012) construction
  arc A366 (113.411, 96.012) -> (112.649, 96.012) centre (113.03, 96.012) ccw construction
  arc A367 (112.649, 94.488) -> (113.411, 94.488) centre (113.03, 94.488) ccw construction
  line L320 (113.03, 94.488) -> (113.03, 96.012) construction
  arc A368 (113.411, 96.012) -> (112.649, 96.012) centre (113.03, 96.012) ccw construction
  arc A369 (112.649, 94.488) -> (113.411, 94.488) centre (113.03, 94.488) ccw construction
  line L321 (115.57, 94.488) -> (115.57, 96.012) construction
  arc A370 (115.951, 96.012) -> (115.189, 96.012) centre (115.57, 96.012) ccw construction
  arc A371 (115.189, 94.488) -> (115.951, 94.488) centre (115.57, 94.488) ccw construction
  line L322 (115.57, 94.488) -> (115.57, 96.012) construction
  arc A372 (115.951, 96.012) -> (115.189, 96.012) centre (115.57, 96.012) ccw construction
  arc A373 (115.189, 94.488) -> (115.951, 94.488) centre (115.57, 94.488) ccw construction
  line L323 (118.11, 94.488) -> (118.11, 96.012) construction
  arc A374 (118.491, 96.012) -> (117.729, 96.012) centre (118.11, 96.012) ccw construction
  arc A375 (117.729, 94.488) -> (118.491, 94.488) centre (118.11, 94.488) ccw construction
  line L324 (118.11, 94.488) -> (118.11, 96.012) construction
  arc A376 (118.491, 96.012) -> (117.729, 96.012) centre (118.11, 96.012) ccw construction
  arc A377 (117.729, 94.488) -> (118.491, 94.488) centre (118.11, 94.488) ccw construction
  line L325 (120.65, 94.488) -> (120.65, 96.012) construction
  arc A378 (121.031, 96.012) -> (120.269, 96.012) centre (120.65, 96.012) ccw construction
  arc A379 (120.269, 94.488) -> (121.031, 94.488) centre (120.65, 94.488) ccw construction
  line L326 (120.65, 94.488) -> (120.65, 96.012) construction
  arc A380 (121.031, 96.012) -> (120.269, 96.012) centre (120.65, 96.012) ccw construction
  arc A381 (120.269, 94.488) -> (121.031, 94.488) centre (120.65, 94.488) ccw construction
  line L327 (123.19, 94.488) -> (123.19, 96.012) construction
  arc A382 (123.571, 96.012) -> (122.809, 96.012) centre (123.19, 96.012) ccw construction
  arc A383 (122.809, 94.488) -> (123.571, 94.488) centre (123.19, 94.488) ccw construction
  line L328 (123.19, 94.488) -> (123.19, 96.012) construction
  arc A384 (123.571, 96.012) -> (122.809, 96.012) centre (123.19, 96.012) ccw construction
  arc A385 (122.809, 94.488) -> (123.571, 94.488) centre (123.19, 94.488) ccw construction
  line L329 (125.73, 94.488) -> (125.73, 96.012) construction
  arc A386 (126.111, 96.012) -> (125.349, 96.012) centre (125.73, 96.012) ccw construction
  arc A387 (125.349, 94.488) -> (126.111, 94.488) centre (125.73, 94.488) ccw construction
  line L330 (125.73, 94.488) -> (125.73, 96.012) construction
  arc A388 (126.111, 96.012) -> (125.349, 96.012) centre (125.73, 96.012) ccw construction
  arc A389 (125.349, 94.488) -> (126.111, 94.488) centre (125.73, 94.488) ccw construction
  line L331 (128.27, 94.488) -> (128.27, 96.012) construction
  arc A390 (128.651, 96.012) -> (127.889, 96.012) centre (128.27, 96.012) ccw construction
  arc A391 (127.889, 94.488) -> (128.651, 94.488) centre (128.27, 94.488) ccw construction
  line L332 (128.27, 94.488) -> (128.27, 96.012) construction
  arc A392 (128.651, 96.012) -> (127.889, 96.012) centre (128.27, 96.012) ccw construction
  arc A393 (127.889, 94.488) -> (128.651, 94.488) centre (128.27, 94.488) ccw construction
  line L333 (130.81, 94.488) -> (130.81, 96.012) construction
  arc A394 (131.191, 96.012) -> (130.429, 96.012) centre (130.81, 96.012) ccw construction
  arc A395 (130.429, 94.488) -> (131.191, 94.488) centre (130.81, 94.488) ccw construction